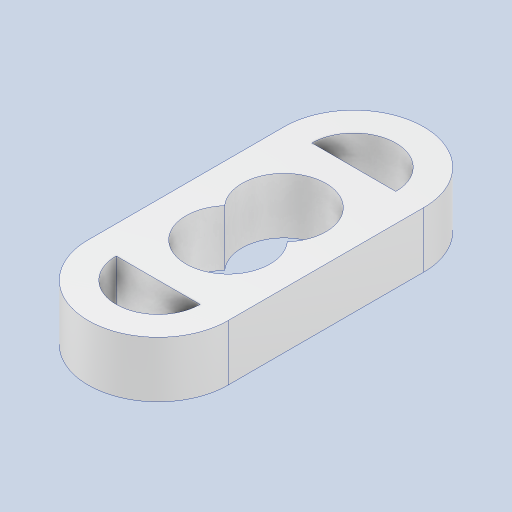
# Autodesk Inventor part: mod4
Saved by Autodesk Inventor 2024 (Build 280153000, 153)
## iProperties
Created: 2025-12-02
Part Number: mod4
Material: Aluminio 6061
Document SubType Name: Modeling
Designer: ANDRES
Density: 2.7 g/cm^3
Appearance: Aluminio - Plano
Author: ANDRES
Autodesk Inventor part; units mm, degrees
ref_plane "YZ Plane" through (0, 0, 0) normal (1, 0, 0) x (0, 1, 0)
ref_plane "XZ Plane" through (0, 0, 0) normal (0, 1, 0) x (-1, 0, 0)
ref_plane "XY Plane" through (0, 0, 0) normal (0, 0, 1) x (1, 0, 0)
sketch "Boceto1" plane through (0, 0, 0) normal (0, 1, 0) x (-1, 0, 0)
  line L0 (0, 35) -> (0, -35) construction
  line L1 (25, 35) -> (25, -35)
  line L2 (-25, -35) -> (-25, 35)
  arc A0 (25, 35) -> (-25, 35) centre (0, 35) ccw
  arc A1 (-25, -35) -> (25, -35) centre (0, -35) ccw
  circle A2 centre (0, -35) radius 15
  circle A3 centre (0, 35) radius 15
  line L3 (0, -20) -> (0, -20)
  line L4 (15, -35) -> (-15, -35)
  line L5 (94.5074, 0) -> (-76.0102, 0) construction
  line L6 (15, 35) -> (-15, 35)
  line L7 (15, -35) -> (-15, -35)
  circle A4 centre (0, 10) radius 15
  circle A5 centre (0, -10) radius 15
  point P0 (0, 0)
  point P1 (0, 60)
  point P2 (0, -60)
  point P3 (0, -20)
  point P4 (15, 35)
  point P5 (11.1803, 0)
  point P6 (-11.1803, 0)
  dimension "largo" = 120
  dimension "ancho" = 50
  dimension "espesor_junta" = 10
  dimension "d3" = 10
  dimension "d6" = 0
  dimension "d22" = 30
  dimension "d23" = 30
  dimension "d24" = 20
  dimension "d25" = 10
  constraints: 18 end point, 10 point on circle, 6 centre point, 4 tangent, 3 horizontal, 3 midpoint, 3 vertical alignment, 2 concentric, 2 symmetric about line, 2 vertical, 1 parallel
  measures "largo" distance of point (0, 60) point (0, -60)
  measures "ancho" distance between parallel lines of L2 L1
  measures "espesor_junta" radial gap between concentric circles of A1 A2
  measures "d3" radial gap between concentric circles of A0 A3
  measures "d6" distance of L3.start L3.end
  measures "d22" diameter of A4
  measures "d23" diameter of A5
  measures "d24" distance of A5.centre A4.centre
  measures "d25" distance of point (0, 0) A5.centre
extrude "Extrusión6" add sketch "Boceto1" along normal blind 20 contours L1 A1 L2 A0 | A2 A5 L4 | A3 L6 A4
equation "\"d3\" = espesor_junta"
